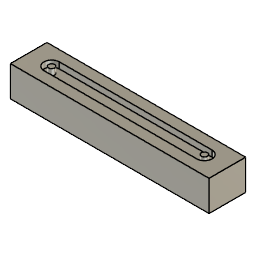
hexbug_5.5cm_mold v1 (Autodesk Fusion 360 design; units mm, degrees)
Autodesk Fusion 360 part; units mm, degrees
note: some values were not read from the file. Set by a fixed rule: which sketch regions a step uses.
sketch "Sketch1" plane through (0, 0, 0) normal (0, 0, 1) x (1, 0, 0)
  line L0 (0, 0) -> (-55, 0)
  line L1 (-55, 0) -> (-55, -12)
  line L2 (-55, -12) -> (0, -12)
  line L3 (0, -12) -> (0, 0)
  dimension "d1" = 12
  dimension "d2" = 55
  constraint horizontal L0
  constraint vertical L1
  constraint horizontal L2
  constraint vertical L3
  constraint coincident L0.start L3.end
  measures "d1" distance of L0.start L2.end
  measures "d2" distance of L0.start L0.end
extrude "Extrude1" add sketch "Sketch1" along normal blind 10
sketch "Sketch2" plane through (0, 0, 10) normal (0, 0, 1) x (-1, 0, 0)
  line L0 (0, 12) -> (0, 0)
  line L1 (0, 0) -> (55, 0)
  line L2 (55, 0) -> (55, 12)
  line L3 (55, 12) -> (0, 12)
  line L4 (0, 6) -> (55, 6)
  line L5 (27.5, 12) -> (27.5, 0)
  line L6 (27.5, 6) -> (2.5, 6)
  line L7 (27.5, 6) -> (52.5, 6)
  circle A0 centre (2.5, 6) radius 1
  circle A1 centre (2.5, 6) radius 2.5
  circle A2 centre (52.5, 6) radius 1
  circle A3 centre (52.5, 6) radius 2.5
  line L8 (2.5, 6) -> (2.5, 3.5)
  line L9 (52.5, 3.5) -> (2.5, 3.5)
  line L10 (2.5, 8.5) -> (52.5, 8.5)
  dimension "d5" = 25
  dimension "d6" = 25
  dimension "d7" = 2
  dimension "d8" = 5
  dimension "d9" = 2
  dimension "d10" = 5
  constraint midpoint L0 L4.start
  constraint midpoint L2 L4.end
  constraint midpoint L3 L5.start
  constraint midpoint L1 L5.end
  constraint midpoint L4 L6.start
  constraint perpendicular L0 L6
  constraint perpendicular L5 L7
  constraint coincident L6.end A0.centre
  constraint concentric A0 A1
  constraint coincident L7.end A2.centre
  constraint concentric A2 A3
  constraint coincident A1 L8.end
  constraint perpendicular L4 L8
  constraint coincident A3 L9.start
  constraint tangent A1 L9
  constraint coincident A1 L10.start
  constraint coincident A3 L10.end
  constraint tangent A3 L10
  constraint parallel L9 L10
  measures "d5" distance of L6.start L6.end
  measures "d6" distance of L6.start L7.end
  measures "d7" diameter of A0
  measures "d8" diameter of A1
  measures "d9" diameter of A2
  measures "d10" diameter of A3
extrude "Extrude2" add 1 faces at (0, -8, 3.3333) along direction (1, 0, 0) blind 5
extrude "Extrude3" add 1 faces at (-55, -4, 3.3333) along direction (-1, 0, 0) blind 5
extrude "Extrude4" cut sketch "Sketch2" against normal blind 2 contours L4 L6 A0 A1 | L4 A0 A1 L8 | L4 L5 L6 A1 L10 | L4 L6 A0 A1 L8 | L4 L5 L6 A1 L9 | L4 L5 L7 A3 L10 | L4 L5 L7 A3 L9 | L4 L7 A2 A3 | L4 L7 A2 A3
